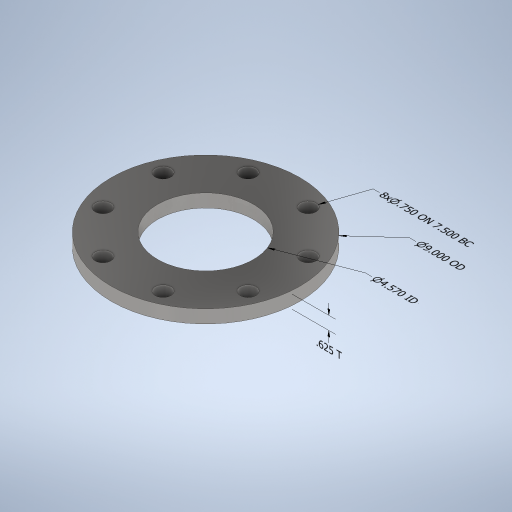
# Autodesk Inventor part: AWWA-C207-B4-S
Saved by Autodesk Inventor 2023 (Build 270158000, 158)
## iProperties
Company: DEMO
RuleStatus: InUse
Created: 2023-06-05
Part Number: AWWA-C207-B4-S
Material: Generic
Document SubType Name: Modeling
Designer: Admin
Density: 1 g/cm^3
Appearance: Steel - Polished
Author: Admin
Autodesk Inventor part; units mm, degrees
ref_plane "YZ Plane" through (0, 0, 0) normal (1, 0, 0) x (0, 1, 0)
ref_plane "XZ Plane" through (0, 0, 0) normal (0, 1, 0) x (-1, 0, 0)
ref_plane "XY Plane" through (0, 0, 0) normal (0, 0, 1) x (1, 0, 0)
sketch "Flange Sketch" plane through (0, 0, 0) normal (0, 1, 0) x (-1, 0, 0)
  circle A0 centre (0, 0) radius 114.3
  circle A1 centre (0, 0) radius 58.039
  circle A2 centre (0, 0) radius 95.25 construction
  line L0 (0, 0) -> (-36.4506, -87.9995) construction
  line L1 (0, 0) -> (0, -95.25) construction
  dimension "outerDiam" = 228.6
  dimension "innerDiam" = 116.078
  dimension "boltCircle" = 190.5
  dimension "boltOffsetAngle" = 22.5
  constraints: 4 end point, 3 centre point, 3 coincident, 2 point on circle, 1 vertical
  measures "outerDiam" diameter of A0
  measures "innerDiam" diameter of A1
  measures "boltCircle" diameter of A2
  measures "boltOffsetAngle" angle of L0 L1
extrude "Flange Extrusion" add sketch "Flange Sketch" along normal blind 15.875
hole "Bolt Hole" at (36.4506, 0, -87.9995) direction (0, 1, 0) diameter 19.05 depth 15.875
pattern_circular "Bolt Hole Pattern" count 8 over 360 about axis through (0, -10, 0) along (0, 1, 0) of "Bolt Hole"
equation "\"nominalSize\" = 101.6"
body "Solid1"
